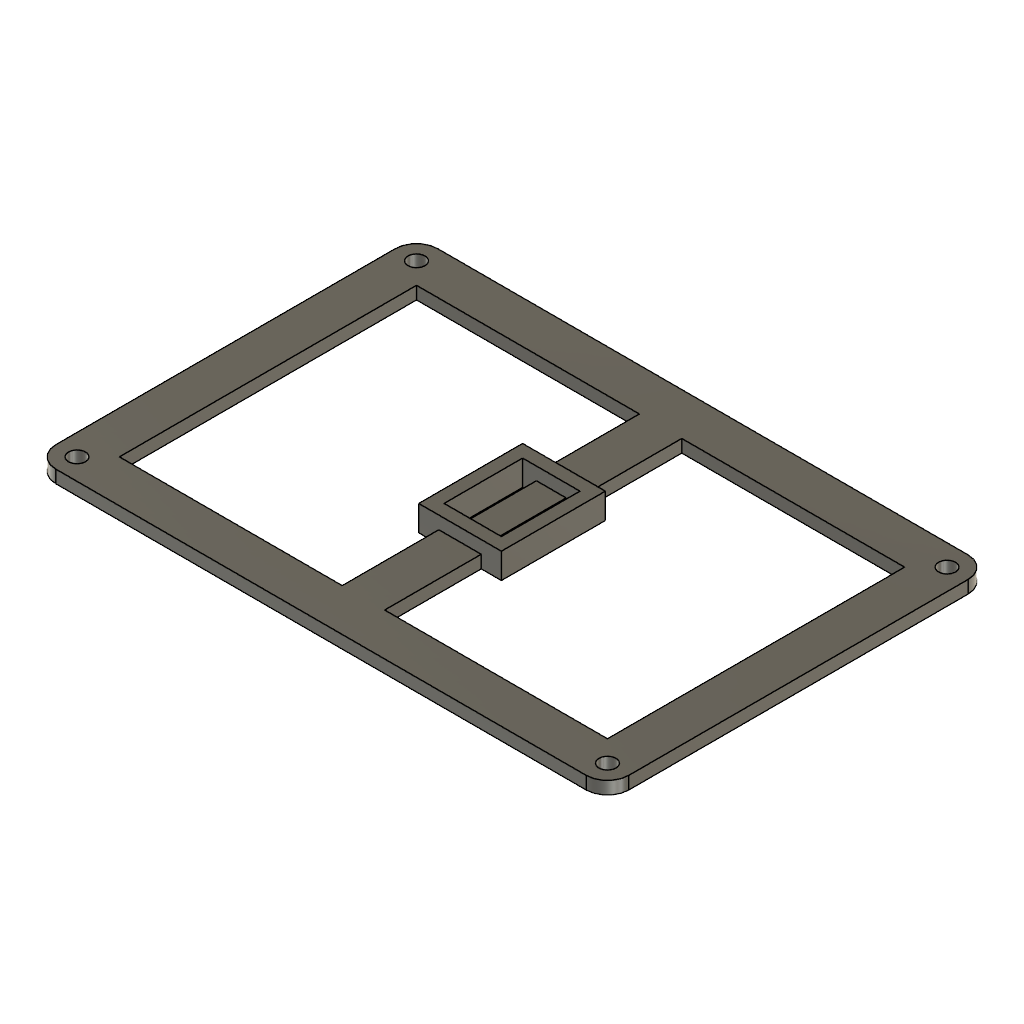
Soporte del Giroscopio_ (Autodesk Fusion 360 design; units mm, degrees)
Autodesk Fusion 360 part; units mm, degrees
note: some values were not read from the file. Set by a fixed rule: which sketch regions a step uses.
sketch "Boceto1" plane through (0, 0, 0) normal (0, 0, 1) x (1, 0, 0)
  line L0 (-6.75, 9.25) -> (6.75, 9.25)
  line L1 (6.75, 9.25) -> (6.75, -9.25)
  line L2 (6.75, -9.25) -> (-6.75, -9.25)
  line L3 (-6.75, -9.25) -> (-6.75, 9.25)
  line L4 (-6.75, 9.25) -> (6.75, -9.25) construction
  line L5 (6.75, 9.25) -> (-6.75, -9.25) construction
  line L6 (9.75, -12.25) -> (-9.75, -12.25)
  line L7 (-9.75, -12.25) -> (-9.75, 12.25)
  line L8 (-9.75, 12.25) -> (9.75, 12.25)
  line L9 (9.75, 12.25) -> (9.75, -12.25)
  line L10 (6.75, 0) -> (3.75, 0) construction
  line L11 (-6.75, 0) -> (-3.75, 0) construction
  line L12 (3.5, 0) -> (-3.5, 0)
  line L13 (-3.5, -9.25) -> (-3.5, 9.25)
  line L14 (3.5, -9.25) -> (3.5, 9.25)
  dimension "d1" = 13.5
  dimension "d2" = 18.5
  dimension "d3" = -3
  dimension "d4" = 3
  dimension "d5" = 3
  dimension "d6" = 7
  constraint horizontal L0
  constraint perpendicular L0 L1
  constraint parallel L0 L2
  constraint parallel L1 L3
  constraint coincident L4 origin
  constraint coincident L5 origin
  constraint midpoint L1 L10.start
  constraint perpendicular L1 L10
  constraint midpoint L3 L11.start
  constraint perpendicular L3 L11
  constraint midpoint L12 origin
  constraint parallel L11 L12
  constraint midpoint L12.end L13
  constraint coincident L0 L13.end
  constraint perpendicular L0 L13
  constraint midpoint L12.start L14
  constraint coincident L0 L14.end
  constraint perpendicular L0 L14
  measures "d1" distance of L1.end L2.end
  measures "d2" distance of L0.end L1.end
  measures "d4" distance of L10.start L10.end
  measures "d5" distance of L11.start L11.end
  measures "d6" distance of L12.start L12.end
extrude "Extruir1" add sketch "Boceto1" along normal blind 6
extrude "Extruir2" add sketch "Boceto1" along normal blind 3 contours L0 L12 L13 L14 | L2 L12 L13 L14
sketch "Boceto2" plane through (0, 0, 0) normal (0, 0, -1) x (1, 0, 0)
  line L0 (-3.5, -9.25) -> (-6.75, -9.25)
  line L1 (-6.75, -9.25) -> (-6.75, 9.25)
  line L2 (-6.75, 9.25) -> (-3.5, 9.25)
  line L3 (-3.5, 9.25) -> (-3.5, -9.25)
  line L4 (3.5, -9.25) -> (3.5, 9.25)
  line L5 (3.5, 9.25) -> (6.75, 9.25)
  line L6 (6.75, 9.25) -> (6.75, -9.25)
  line L7 (6.75, -9.25) -> (3.5, -9.25)
  line L8 (-9.75, -12.25) -> (9.75, -12.25)
  line L9 (9.75, -12.25) -> (9.75, 12.25)
  line L10 (9.75, 12.25) -> (-9.75, 12.25)
  line L11 (-9.75, 12.25) -> (-9.75, -12.25)
  line L12 (-67.5, 45) -> (67.5, 45)
  line L13 (67.5, 45) -> (67.5, -45)
  line L14 (67.5, -45) -> (-67.5, -45)
  line L15 (-67.5, -45) -> (-67.5, 45)
  line L16 (-67.5, 45) -> (67.5, -45) construction
  line L17 (67.5, 45) -> (-67.5, -45) construction
  line L18 (-67.5, 45) -> (-62.5, 45)
  line L19 (-62.5, 45) -> (-62.5, 40)
  line L20 (-67.5, -45) -> (-62.5, -45)
  line L21 (-62.5, -45) -> (-62.5, -40)
  line L22 (67.5, -45) -> (62.5, -45)
  line L23 (62.5, -45) -> (62.5, -40)
  line L24 (67.5, 45) -> (62.5, 45)
  line L25 (62.5, 45) -> (62.5, 40)
  circle A0 centre (-62.5, 40) radius 2
  circle A1 centre (-62.5, -40) radius 2
  circle A2 centre (62.5, -40) radius 2
  circle A3 centre (62.5, 40) radius 2
  line L26 (0, -12.25) -> (0, -40)
  line L27 (0, 12.25) -> (0, 40)
  line L28 (-62.5, -40) -> (-62.5, 40) construction
  line L29 (62.5, -40) -> (62.5, 40) construction
  circle A4 centre (-62.5, 40) radius 5
  circle A5 centre (62.5, 40) radius 5
  circle A6 centre (-62.5, -40) radius 5
  circle A7 centre (62.5, -40) radius 5
  line L30 (5, -40) -> (-5, -40)
  line L31 (5, 40) -> (-5, 40)
  line L32 (-5, 40) -> (-5, 12.25)
  line L33 (5, 40) -> (5, 12.25)
  line L34 (-5, -40) -> (-5, -12.25)
  line L35 (5, -40) -> (5, -12.25)
  line L36 (-62.5, -45) -> (62.5, -45)
  arc A8 (62.5, -45) -> (62.5, -35) centre (62.5, -40) ccw
  line L37 (62.5, -35) -> (-62.5, -35)
  arc A9 (-62.5, -35) -> (-62.5, -45) centre (-62.5, -40) ccw
  line L38 (-62.5, -40) -> (62.5, -40) construction
  line L39 (-62.5, 35) -> (62.5, 35)
  arc A10 (62.5, 35) -> (62.5, 45) centre (62.5, 40) ccw
  line L40 (62.5, 45) -> (-62.5, 45)
  arc A11 (-62.5, 45) -> (-62.5, 35) centre (-62.5, 40) ccw
  line L41 (-62.5, 40) -> (62.5, 40) construction
  line L42 (-57.5, -40) -> (-57.5, 40)
  arc A12 (-57.5, 40) -> (-67.5, 40) centre (-62.5, 40) ccw
  line L43 (-67.5, 40) -> (-67.5, -40)
  arc A13 (-67.5, -40) -> (-57.5, -40) centre (-62.5, -40) ccw
  line L44 (-62.5, -40) -> (-62.5, 40) construction
  line L45 (67.5, -40) -> (67.5, 40)
  arc A14 (67.5, 40) -> (57.5, 40) centre (62.5, 40) ccw
  line L46 (57.5, 40) -> (57.5, -40)
  arc A15 (57.5, -40) -> (67.5, -40) centre (62.5, -40) ccw
  line L47 (62.5, -40) -> (62.5, 40) construction
  dimension "d11" = 135
  dimension "d12" = 90
  dimension "d13" = 5
  dimension "d14" = 5
  dimension "d15" = 5
  dimension "d16" = 5
  dimension "d17" = 5
  dimension "d18" = 5
  dimension "d19" = 5
  dimension "d20" = 5
  dimension "d21" = 4
  dimension "d22" = 4
  dimension "d23" = 4
  dimension "d24" = 4
  dimension "d25" = 10
  dimension "d26" = 10
  dimension "d27" = 10
  dimension "d28" = 10
  dimension "d29" = 10
  dimension "d30" = 10
  dimension "d31" = 10
  dimension "d32" = 10
  constraint horizontal L12
  constraint perpendicular L12 L13
  constraint parallel L12 L14
  constraint parallel L13 L15
  constraint coincident L16 origin
  constraint coincident L17 origin
  constraint perpendicular L15 L18
  constraint perpendicular L18 L19
  constraint perpendicular L15 L20
  constraint perpendicular L20 L21
  constraint perpendicular L13 L22
  constraint perpendicular L22 L23
  constraint perpendicular L13 L24
  constraint perpendicular L12 L25
  constraint coincident L19.end A0.centre
  constraint coincident L21.end A1.centre
  constraint coincident L23.end A2.centre
  constraint coincident L25.end A3.centre
  constraint midpoint L8 L26.start
  constraint perpendicular L14 L26
  constraint midpoint L10 L27.start
  constraint perpendicular L10 L27
  constraint concentric A0 A4
  constraint concentric A3 A5
  constraint concentric A1 A6
  constraint concentric A2 A7
  constraint midpoint L26.end L30
  constraint perpendicular L26 L30
  constraint midpoint L27.end L31
  constraint perpendicular L27 L31
  constraint coincident L10 L32.end
  constraint perpendicular L2 L32
  constraint coincident L10 L33.end
  constraint perpendicular L10 L33
  constraint coincident L8 L34.end
  constraint perpendicular L8 L34
  constraint coincident L8 L35.end
  constraint perpendicular L8 L35
  constraint tangent L36 A8
  constraint tangent A8 L37
  constraint parallel L36 L37
  constraint tangent L37 A9
  constraint tangent L36 A9
  constraint perpendicular L23 L38
  constraint tangent L39 A10
  constraint tangent A10 L40
  constraint parallel L39 L40
  constraint tangent L40 A11
  constraint tangent L39 A11
  constraint perpendicular L29 L41
  constraint tangent L42 A12
  constraint tangent A12 L43
  constraint parallel L42 L43
  constraint tangent L43 A13
  constraint tangent L42 A13
  constraint perpendicular L41 L44
  constraint tangent L45 A14
  constraint tangent A14 L46
  constraint parallel L45 L46
  constraint tangent L46 A15
  constraint tangent L45 A15
  constraint perpendicular L41 L47
  measures "d29" distance of L30.start L30.end
  measures "d30" distance of L31.start L31.end
extrude "Extruir3" add sketch "Boceto2" against normal blind 3 contours L8 L26 L34 L37 | L8 L26 L35 L37 | L26 L30 L34 L37 | L14 A6 A7 L30 L34 L35 L36 L37 L42 A13 L46 A15 | L10 L27 L32 L39 | L26 L30 L35 L37 | A6 L37 L42 | L15 A4 A6 L37 A9 L39 A11 L42 L43 | L10 L27 L33 L39 | L12 A4 A5 L31 L32 L33 L39 L40 L42 A12 A14 L46 | L27 L31 L32 L39 | A6 A9 A13 | A4 L39 L42 | L27 L31 L33 L39 | L13 A5 A7 A8 L37 L39 A10 L45 L46 | A7 L37 L46 | A4 A11 A12 | A7 A8 A15 | A5 L39 L46 | A5 A10 A14
